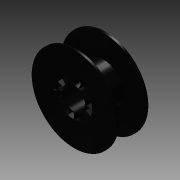
# Autodesk Inventor part: SpoolFilament
Saved by Autodesk Inventor 2015 SP1 (Build 190203100, 203)
## iProperties
Created: 2014-05-26
Part Number: SpoolFilament
Material: ABS Plastic
Document SubType Name: Modeling
Designer: Jack
Density: 1.06 g/cm^3
Appearance: Smooth - Black
Mass: 387.035 g
Surface Area: 1903.77 cm^2
Volume: 365.127 cm^3
Author: Jack
Title: Filament Spool
Autodesk Inventor part; units mm, degrees
ref_plane "YZ Plane" through (0, 0, 0) normal (1, 0, 0) x (0, 1, 0)
ref_plane "XZ Plane" through (0, 0, 0) normal (0, 1, 0) x (-1, 0, 0)
ref_plane "XY Plane" through (0, 0, 0) normal (0, 0, 1) x (1, 0, 0)
sketch "Sketch1" plane through (0, 0, 0) normal (0, 1, 0) x (-1, 0, 0)
  circle A0 centre (0, 0) radius 100
  dimension "d4" = 200
  constraints: 1 centre point, 1 coincident
  measures "d4" diameter of A0
extrude "Extrusion1" add sketch "Sketch1" along normal blind 5
sketch "Sketch2" plane through (0, 5, 0) normal (0, 1, 0) x (1, 0, 0)
  circle A0 centre (0, 0) radius 100 projected
  circle A1 centre (0, 0) radius 45.75
  dimension "d7" = 91.5
  constraints: 1 centre point, 1 coincident
  measures "d7" diameter of A1
extrude "Extrusion2" add sketch "Sketch2" along normal blind 64 contours A1
sketch "Sketch3" plane through (0, 69, 0) normal (0, 1, 0) x (1, 0, 0)
  circle A0 centre (0, 0) radius 45.75 projected
  circle A1 centre (0, 0) radius 100
  dimension "d10" = 200
  constraints: 1 centre point, 1 coincident
  measures "d10" diameter of A1
extrude "Extrusion3" add sketch "Sketch3" along normal blind 5 contours A0 | A1
sketch "Sketch4" plane through (0, 74, 0) normal (0, 1, 0) x (1, 0, 0)
  circle A0 centre (0, 0) radius 100 projected
  circle A1 centre (0, 0) radius 42
  dimension "d13" = 84
  constraints: 1 centre point, 1 coincident
  measures "d13" diameter of A1
extrude "Extrusion4" cut sketch "Sketch4" against normal up to surface (74 mm away) contours A1
sketch "Sketch5" plane through (0, 0, 0) normal (0, -1, 0) x (1, 0, 0)
  circle A0 centre (0, 0) radius 100 projected
  circle A1 centre (0, 0) radius 25.75
  circle A2 centre (0, 0) radius 28.3
  dimension "d16" = 51.5
  dimension "d17" = 56.6
  constraints: 2 centre point, 2 coincident
  measures "d16" diameter of A1
  measures "d17" diameter of A2
extrude "Extrusion5" add sketch "Sketch5" against normal up to surface (74 mm away) contours A2
sketch "Sketch7" plane through (0, 0, 0) normal (0, -1, 0) x (1, 0, 0)
  circle A0 centre (0, 0) radius 25.75 projected
  circle A1 centre (0, 0) radius 28.3 projected
  line L0 (28.2936, 0.6) -> (41.9957, 0.6)
  circle A2 centre (0, 0) radius 42 projected
  line L1 (28.2936, -0.6) -> (41.9957, -0.6)
  dimension "d21" = 1.2
  dimension "d22" = 0.6
  constraints: 4 end point, 4 point on circle, 2 horizontal
  measures "d21" distance between parallel lines of L0 L1
  measures "d22" vertical distance of A0.centre L1.start
extrude "Extrusion6" add sketch "Sketch7" against normal up to surface (74 mm away) contours A1 L0 A2 L1 picked at (32.8649, -0.3333)
pattern_circular "Circular Pattern1" count 16 over 360 about axis through (0, 0, 0) along (0, 1, 0) of "Extrusion6"
sketch "Sketch8" plane through (0, 74, 0) normal (0, 1, 0) x (1, 0, 0)
  arc A0 (26.3695, -10.2732) -> (28.2936, -0.6) centre (0, 0) ccw projected
  circle A1 centre (0, 0) radius 25.75 projected
  circle A2 centre (-44.25, 0) radius 5.25
  circle A3 centre (0, 0) radius 25.75 projected
  point P0 (25.75, 0)
  dimension "d28" = 10.5
  dimension "d29" = 70
  constraints: 4 horizontal alignment, 1 centre point, 2 other
  measures "d28" diameter of A2
  measures "d29" distance of A2.centre point (25.75, 0)
extrude "Extrusion7" cut sketch "Sketch8" against normal blind 3.6 contours A2
sketch "Sketch9" plane through (0, 0, 0) normal (0, -1, 0) x (1, 0, 0)
  arc A0 (25.9103, 11.3818) -> (20.4309, 19.5824) centre (0, 0) ccw projected
  circle A1 centre (0, 0) radius 25.75 projected
  circle A2 centre (-44.25, 0) radius 5.25
  circle A3 centre (0, 0) radius 25.75 projected
  point P0 (25.75, 0)
  dimension "d32" = 10.5
  dimension "d34" = 70
  constraints: 4 horizontal alignment, 1 centre point, 2 other
  measures "d32" diameter of A2
  measures "d34" distance of A2.centre point (25.75, 0)
extrude "Extrusion8" cut sketch "Sketch9" against normal blind 3.6 contours A2
sketch "Sketch10" plane through (0, 74, 0) normal (0, 1, 0) x (1, 0, 0)
  line L0 (39.0286, 15.5167) -> (26.3695, 10.2732) projected
  arc A0 (41.9957, 0.6) -> (39.0286, 15.5167) centre (0, 0) ccw projected
  line L1 (28.2936, 0.6) -> (41.9957, 0.6) projected
  arc A1 (28.2936, 0.6) -> (26.3695, 10.2732) centre (0, 0) ccw projected
  circle A2 centre (0, 0) radius 25.75 projected
  line L2 (30.1197, 29.2712) -> (20.4309, 19.5824) projected
  arc A3 (38.5694, 16.6254) -> (30.1197, 29.2712) centre (0, 0) ccw projected
  line L3 (25.9103, 11.3818) -> (38.5694, 16.6254) projected
  arc A4 (25.9103, 11.3818) -> (20.4309, 19.5824) centre (0, 0) ccw projected
  line L4 (16.6254, 38.5694) -> (11.3818, 25.9103) projected
  arc A5 (29.2712, 30.1197) -> (16.6254, 38.5694) centre (0, 0) ccw projected
  line L5 (19.5824, 20.4309) -> (29.2712, 30.1197) projected
  arc A6 (19.5824, 20.4309) -> (11.3818, 25.9103) centre (0, 0) ccw projected
  line L6 (0.6, 41.9957) -> (0.6, 28.2936) projected
  arc A7 (15.5167, 39.0286) -> (0.6, 41.9957) centre (0, 0) ccw projected
  line L7 (10.2732, 26.3695) -> (15.5167, 39.0286) projected
  arc A8 (10.2732, 26.3695) -> (0.6, 28.2936) centre (0, 0) ccw projected
  line L8 (-15.5167, 39.0286) -> (-10.2732, 26.3695) projected
  arc A9 (-0.6, 41.9957) -> (-15.5167, 39.0286) centre (0, 0) ccw projected
  line L9 (-0.6, 28.2936) -> (-0.6, 41.9957) projected
  arc A10 (-0.6, 28.2936) -> (-10.2732, 26.3695) centre (0, 0) ccw projected
  line L10 (-29.2712, 30.1197) -> (-19.5824, 20.4309) projected
  arc A11 (-16.6254, 38.5694) -> (-29.2712, 30.1197) centre (0, 0) ccw projected
  line L11 (-11.3818, 25.9103) -> (-16.6254, 38.5694) projected
  arc A12 (-11.3818, 25.9103) -> (-19.5824, 20.4309) centre (0, 0) ccw projected
  line L12 (-38.5694, 16.6254) -> (-25.9103, 11.3818) projected
  arc A13 (-30.1197, 29.2712) -> (-38.5694, 16.6254) centre (0, 0) ccw projected
  line L13 (-20.4309, 19.5824) -> (-30.1197, 29.2712) projected
  arc A14 (-20.4309, 19.5824) -> (-25.9103, 11.3818) centre (0, 0) ccw projected
  line L14 (-30.1197, -29.2712) -> (-20.4309, -19.5824) projected
  arc A15 (-38.5694, -16.6254) -> (-30.1197, -29.2712) centre (0, 0) ccw projected
  line L15 (-25.9103, -11.3818) -> (-38.5694, -16.6254) projected
  arc A16 (-25.9103, -11.3818) -> (-20.4309, -19.5824) centre (0, 0) ccw projected
  line L16 (-16.6254, -38.5694) -> (-11.3818, -25.9103) projected
  arc A17 (-29.2712, -30.1197) -> (-16.6254, -38.5694) centre (0, 0) ccw projected
  line L17 (-19.5824, -20.4309) -> (-29.2712, -30.1197) projected
  arc A18 (-19.5824, -20.4309) -> (-11.3818, -25.9103) centre (0, 0) ccw projected
  line L18 (-0.6, -41.9957) -> (-0.6, -28.2936) projected
  arc A19 (-15.5167, -39.0286) -> (-0.6, -41.9957) centre (0, 0) ccw projected
  line L19 (-10.2732, -26.3695) -> (-15.5167, -39.0286) projected
  arc A20 (-10.2732, -26.3695) -> (-0.6, -28.2936) centre (0, 0) ccw projected
  line L20 (15.5167, -39.0286) -> (10.2732, -26.3695) projected
  arc A21 (0.6, -41.9957) -> (15.5167, -39.0286) centre (0, 0) ccw projected
  line L21 (0.6, -28.2936) -> (0.6, -41.9957) projected
  arc A22 (0.6, -28.2936) -> (10.2732, -26.3695) centre (0, 0) ccw projected
  line L22 (29.2712, -30.1197) -> (19.5824, -20.4309) projected
  arc A23 (16.6254, -38.5694) -> (29.2712, -30.1197) centre (0, 0) ccw projected
  line L23 (11.3818, -25.9103) -> (16.6254, -38.5694) projected
  arc A24 (11.3818, -25.9103) -> (19.5824, -20.4309) centre (0, 0) ccw projected
  line L24 (38.5694, -16.6254) -> (25.9103, -11.3818) projected
  arc A25 (30.1197, -29.2712) -> (38.5694, -16.6254) centre (0, 0) ccw projected
  line L25 (20.4309, -19.5824) -> (30.1197, -29.2712) projected
  arc A26 (20.4309, -19.5824) -> (25.9103, -11.3818) centre (0, 0) ccw projected
  arc A27 (26.3695, -10.2732) -> (28.2936, -0.6) centre (0, 0) ccw projected
  line L26 (41.9957, -0.6) -> (28.2936, -0.6) projected
  arc A28 (39.0286, -15.5167) -> (41.9957, -0.6) centre (0, 0) ccw projected
  line L27 (26.3695, -10.2732) -> (39.0286, -15.5167) projected
  circle A29 centre (0, 0) radius 42
  constraints: 1 coincident, 3 other
extrude "Extrusion9" cut sketch "Sketch10" against normal blind 15.5 contours L0 A1 L1 A29 L26 A27 L27 L24 A26 L25 L22 A24 L23 L20 A22 L21 L18 A20 L19 L16 A18 L17 L14 A16 L15 L12 A14 L13 L10 A12 L11 L8 A10 L9 L6 A8 L7 L4 A6 L5 L2 A4 L3
body "Solid1"
